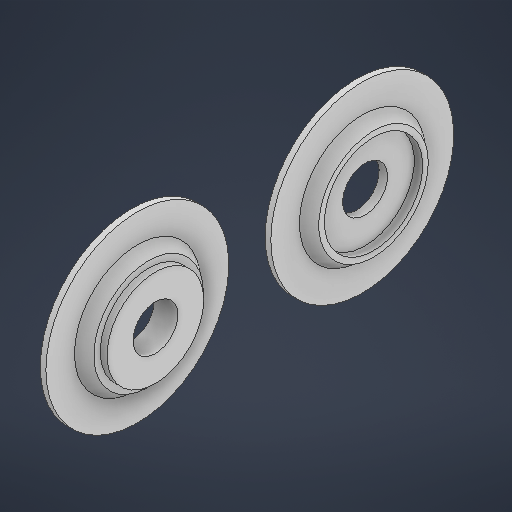
# Autodesk Inventor part: poleas_v13
Saved by Autodesk Inventor 2026.1 (Build 301233020, 233B)
## iProperties
Created: 2026-02-22
Part Number: poleas_v13
Material: Generic
Document SubType Name: Modeling
Designer: user
Density: 1 g/cm^3
Appearance: Default
Author: user
Autodesk Inventor part; units mm, degrees
ref_plane "YZ Plane" through (0, 0, 0) normal (1, 0, 0) x (0, 1, 0)
ref_plane "XZ Plane" through (0, 0, 0) normal (0, 1, 0) x (-1, 0, 0)
ref_plane "XY Plane" through (0, 0, 0) normal (0, 0, 1) x (1, 0, 0)
sketch "Sketch1" plane through (0, 0, 0) normal (1, 0, 0) x (0, 1, 0)
  circle A0 centre (0, 0) radius 4.8704
  dimension "d0" = 9.7409
  constraints: 1 centre point, 1 coincident
  measures "d0" diameter of A0
extrude "Extrusion1" add sketch "Sketch1" along normal mid plane 2
sketch "Sketch2" plane through (-1, 0, 0) normal (-1, 0, 0) x (0, 0, 1)
  circle A0 centre (0, 0) radius 8.1325
  constraints: 1 centre point, 1 coincident
extrude "Extrusion2" add sketch "Sketch2" along normal blind 0.5
sketch "Sketch3" plane through (-1.5, 0, 0) normal (-1, 0, 0) x (0, 0, 1)
  point P0 (0, 0)
sketch "Sketch5" plane through (0, 0, 0) normal (0, 1, 0) x (-1, 0, 0)
  circle A0 centre (0, -0.6447) radius 0.3263
  line L0 (-1.5, 0) -> (1.5, 0)
  circle A1 centre (0, 0.6447) radius 0.3263
  point P0 (0, 0)
  constraints: 2 centre point, 2 end point, 1 symmetric about line, 1 other
sketch "Sketch6" plane through (0, 0, 0) normal (0, 1, 0) x (-1, 0, 0)
  line L0 (1, -4.8704) -> (1, 4.8704) projected
  line L1 (1, -4.8704) -> (-1, -4.8704) projected
  line L2 (0, -4.8704) -> (1, -5.5929)
  line L3 (1, -8.1325) -> (1, 8.1325) projected
  line L4 (0, -4.8704) -> (-1, -5.5929)
  line L5 (-1, -5.5929) -> (-1, -4.8704)
  line L6 (1, -4.8704) -> (1, -5.5929)
  line L7 (-2.6263, 0) -> (3.0126, 0)
  line L8 (-1, -5.5929) -> (-1, -4.8704)
  line L9 (0, -4.8704) -> (1, -4.8704)
  point P0 (0, 0)
  constraints: 14 end point, 1 horizontal, 1 midpoint, 1 perpendicular, 1 point on line
revolve "Revolution1" add sketch "Sketch6" angle 360 about axis through (2.6263, 0, 0) along (-1, 0, 0)
sketch "Sketch7" plane through (0, 0, 0) normal (0, 1, 0) x (-1, 0, 0)
  line L0 (-5.9098, -5.7705) -> (0, -5.7705)
  line L1 (0, -5.7705) -> (0, 6.7499)
  line L2 (0, 6.7499) -> (-5.9098, 6.7499)
  line L3 (-5.9098, 6.7499) -> (-5.9098, -5.7705)
  point P0 (0, 0)
  constraints: 8 end point, 2 parallel, 1 horizontal, 1 perpendicular
extrude "Extrusion6" cut sketch "Sketch7" along normal mid plane 15.75
sketch "Sketch8" plane through (0, 0, 0) normal (1, 0, 0) x (0, 1, 0)
  circle A0 centre (0, 0) radius 2
  dimension "d15" = 4
  constraints: 1 centre point, 1 coincident
  measures "d15" diameter of A0
extrude "Extrusion7" cut sketch "Sketch8" against normal through all
sketch "Sketch9" plane through (0, 0, 0) normal (1, 0, 0) x (0, 0, 1)
  circle A0 centre (0, 0) radius 4.374
  circle A1 centre (0, 0) radius 2 projected
  arc A2 (1.4796, -1.3457) -> (-1.4796, -1.3457) centre (0, 0) ccw
  line L0 (0.971, 0) -> (0.971, -2) projected
  line L1 (-0.971, -2) -> (-0.971, 0) projected
  point P0 (-4.8704, 0)
  point P1 (0, -2)
  point P2 (0, -2)
  point P3 (-4.8704, 0)
  dimension "d36" = 8.7479
  constraints: 3 point on circle, 2 centre point, 2 coincident, 2 other
  measures "d36" diameter of A0
extrude "Extrusion8" cut sketch "Sketch9" against normal blind 0.75 contours A0 | A1
pattern_linear "Rectangular Pattern3" count 2 spacing 20 along (0, 0, 1) of "Extrusion1", "Extrusion2", "Revolution1", "Extrusion6", "Extrusion7"
sketch "Sketch10" plane through (0, 0, 15.1296) normal (1, 0, 0) x (0, 0, -1)
  arc A0 (-4.8704, 2) -> (-4.8704, 2) centre (-4.8704, 0) ccw projected
  circle A1 centre (-4.8704, 0) radius 2
  circle A2 centre (-4.8704, 0) radius 4.299
  point P0 (15.1296, 0)
  dimension "d43" = 8.5979
  constraints: 2 centre point, 2 coincident, 1 concentric
  measures "d43" diameter of A2
extrude "Extrusion9" add sketch "Sketch10" along normal blind 0.6
sketch "Sketch13" plane through (0, 0, 0) normal (1, 0, 0) x (0, 0, -1)
  line L0 (-10.5789, 11.9796) -> (10.4116, 11.9796)
  line L1 (10.4116, 11.9796) -> (10.4116, -10.5162)
  line L2 (10.4116, -10.5162) -> (-10.5789, -10.5162)
  line L3 (-10.5789, -10.5162) -> (-10.5789, 11.9796)
  point P0 (0, 0)
  constraints: 8 end point, 2 parallel, 1 horizontal, 1 perpendicular
sketch "Sketch12" plane through (0.6, 0, 20) normal (1, 0, 0) x (0, 0, -1)
  line L0 (-15.4581, 11.9378) -> (10.0065, 11.9378)
  line L1 (10.0065, 11.9378) -> (10.0065, -10.3907)
  line L2 (10.0065, -10.3907) -> (-15.4581, -10.3907)
  line L3 (-15.4581, -10.3907) -> (-15.4581, 11.9378)
  point P0 (20, 0)
  constraints: 8 end point, 2 parallel, 1 horizontal, 1 perpendicular
sketch "Sketch11" plane through (0, 0, 20) normal (1, 0, 0) x (0, 1, 0)
  line L0 (12.8492, -9.7207) -> (-12.5468, -9.7207)
  line L1 (-12.5468, -9.7207) -> (-12.5468, -34.2097)
  line L2 (-12.5468, -34.2097) -> (12.8492, -34.2097)
  line L3 (12.8492, -34.2097) -> (12.8492, -9.7207)
  point P0 (0, -20)
  constraints: 8 end point, 2 parallel, 1 horizontal, 1 perpendicular
ref_plane "Work Plane7" through (0, 0, 20) normal (1, 0, 0) x (0, 1, 0)
equation "\"tolerancia\" = 0.15"
body "Solid1"
